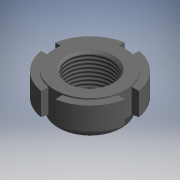
# Autodesk Inventor part: 717739 GUK M10x0.75
Saved by Autodesk Inventor 2017.3 (Build 213256000, 256)
## iProperties
Part Number: 717739 GUK M10x0.75
Material: Generic
Catalog Web Link: www.cadenas.de
Description: GUK-slotted round nut
Vendor: FESTO
Document SubType Name: Modeling
Designer: partserver
Manufacturer: FESTO
Mass: 1.08127 g
Surface Area: 9.61476 cm^2
Volume: 1.08127 cm^3
Density: 1 g/cm^3
Appearance: PSOLRGB-128-128-128
Category: PARTsolutions
Company: FESTO
Title: 717739 GUK M10x0.75
Author: Cadenas PARTsolutions
Comments: slotted round nut
PSOL_IDENT_0: {$CADENAS_DATA\23d-libs\festo\parts\g\guk\guk.prj},175 {VTYP=3D},{NB=717739 GUK M10x0.75},{LINA=7177
PSOL_IDENT_1: 39 GUK M10x0.75},{NN=GUK},{DATE=09.09.2015 14:14:39},{GEOMDATE=03.09.2015 07:34:17},{VERSION=},{LINE
PSOL_IDENT_2: ID=10},{WBVAR=},{WBNUMERIC=}  {NB=717739 GUK M10x0.75},{LINA=717739 GUK M10x0.75},{KT=DUMMY},{TNR=71
PSOL_IDENT_3: 7739},{TYP=GUK},{D=M10x0.75},{DN=10.000},{B=7.600},{B1=0.000},{D1=18.000},{D2=14.900},{A=15.000},{T=
PSOL_IDENT_4: 15.000},{C=3.000},{H=7.600},{P=0.750}
NB: 717739 GUK M10x0.75
NN: GUK
NT: slotted round nut
NBSYN: $TNR. $TYP. $D.
LINA: 717739 GUK M10x0.75
CATALOG: Festo
TNR: 717739
TYP: GUK
D: M10x0.75
DN: 10
B: 7.6
B1: 0
D1: 18
D2: 14.9
A: 15
T: 15
C: 3
H: 7.6
P: 0.75
SUPPLIER: FESTO
ARTICLENO: 717739 GUK M10x0.75
BOMINFO: 717739 GUK M10x0.75
CREATOR: CADENAS GmbH
Autodesk Inventor part; units mm, degrees
sketch "Skizze_1" plane through (0, 0, 0) normal (1, 0, 0) x (0, 1, 0)
  line L0 (0, 0) -> (0, 7.6)
  line L1 (6.2894, 7.6) -> (5, 7.6)
  line L2 (5, 7.6) -> (4.594, 7.194)
  line L3 (4.594, 7.194) -> (4.594, 0.406)
  line L4 (4.594, 0.406) -> (5, 0)
  line L5 (5, 0) -> (7.5, 0)
  line L6 (7.5, 0) -> (7.5, 0.3)
  line L7 (7.5, 0.3) -> (9, 0.3)
  line L8 (9, 0.3) -> (9, 5.1)
  line L9 (9, 5.1) -> (7.45, 5.3733)
  line L10 (7.45, 5.3733) -> (6.7593, 7.271)
  arc A0 (6.7593, 7.271) -> (6.2894, 7.6) centre (6.2894, 7.1) ccw
  constraints: 22 end point, 2 point on circle, 1 centre point
revolve "Revolution1" add sketch "Skizze_1" angle 360 about axis through (0, 0, 0) along (0, 0, -1)
thread "Thread1" size "M10x0.75" class "6H" standard "ISO Metric profile" full length
sketch "Skizze_2" plane through (0, 0, 0) normal (0, 0, 1) x (1, 0, 0)
  line L0 (-18, 18) -> (-18, -18)
  line L1 (-18, -18) -> (18, -18)
  line L2 (18, -18) -> (18, 18)
  line L3 (18, 18) -> (-18, 18)
  arc A0 (-9.8869, -1.5) -> (-1.5, -9.8869) centre (0, 0) ccw
  line L4 (-1.5, -9.8869) -> (-1.5, -7.3485)
  arc A1 (-1.5, -7.3485) -> (1.5, -7.3485) centre (0, 0) ccw
  line L5 (1.5, -7.3485) -> (1.5, -9.8869)
  arc A2 (1.5, -9.8869) -> (9.8869, -1.5) centre (0, 0) ccw
  line L6 (9.8869, -1.5) -> (7.3485, -1.5)
  arc A3 (7.3485, -1.5) -> (7.3485, 1.5) centre (0, 0) ccw
  line L7 (7.3485, 1.5) -> (9.8869, 1.5)
  arc A4 (9.8869, 1.5) -> (1.5, 9.8869) centre (0, 0) ccw
  line L8 (1.5, 9.8869) -> (1.5, 7.3485)
  arc A5 (1.5, 7.3485) -> (-1.5, 7.3485) centre (0, 0) ccw
  line L9 (-1.5, 7.3485) -> (-1.5, 9.8869)
  arc A6 (-1.5, 9.8869) -> (-9.8869, 1.5) centre (0, 0) ccw
  line L10 (-9.8869, 1.5) -> (-7.3485, 1.5)
  arc A7 (-7.3485, 1.5) -> (-7.3485, -1.5) centre (0, 0) ccw
  line L11 (-7.3485, -1.5) -> (-9.8869, -1.5)
  constraints: 24 end point, 16 point on circle, 8 centre point
extrude "Extrusion1" cut sketch "Skizze_2" along normal blind 7.6
ref_plane "ANBAU_XY" through (0, 0, 0) normal (0, 0, 1) x (1, 0, 0)
ref_plane "ANBAU_YZ" through (0, 0, 0) normal (1, 0, 0) x (0, 1, 0)
ref_plane "ANBAU_ZX" through (0, 0, 0) normal (0, 1, 0) x (0, 0, 1)
body "Solid1"
